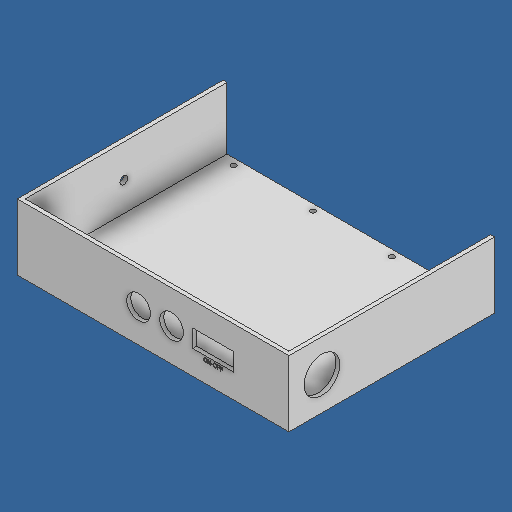
# Autodesk Inventor part: Chasis
Saved by Autodesk Inventor 2025 (Build 290162000, 162)
## iProperties
Created: 2025-09-23
Part Number: Chasis
Material: Genérico
Document SubType Name: Modeling
Designer: HP
Density: 1 g/cm^3
Appearance: Valor por defecto
Author: HP
Autodesk Inventor part; units mm, degrees
ref_plane "YZ Plane" through (0, 0, 0) normal (1, 0, 0) x (0, 1, 0)
ref_plane "XZ Plane" through (0, 0, 0) normal (0, 1, 0) x (-1, 0, 0)
ref_plane "XY Plane" through (0, 0, 0) normal (0, 0, 1) x (1, 0, 0)
sketch "Boceto1" plane through (0, 0, 0) normal (0, 1, 0) x (-1, 0, 0)
  line L0 (-100, 75) -> (100, 75)
  line L1 (100, 75) -> (100, -75)
  line L2 (100, -75) -> (-100, -75)
  line L3 (-100, -75) -> (-100, 75)
  line L4 (-100, 75) -> (100, -75) construction
  line L5 (100, 75) -> (-100, -75) construction
  point P0 (0, 0)
  dimension "d0" = 200
  dimension "d1" = 150
  constraints: 12 end point, 2 midpoint, 2 parallel, 1 horizontal, 1 perpendicular
  measures "d0" distance of L1.end L2.end
  measures "d1" distance of L0.end L1.end
extrude "Extrusión1" add sketch "Boceto1" along normal blind 3
sketch "Boceto2" plane through (0, 0, 0) normal (0, 1, 0) x (-1, 0, 0)
  line L0 (-100, -75) -> (100, -75) projected
  line L1 (100, -75) -> (100, 75) projected
  line L2 (100, 75) -> (-100, 75) projected
  line L3 (-100, 75) -> (-100, -75) projected
  line L4 (103, 78) -> (103, -78)
  line L5 (103, -78) -> (-103, -78)
  line L6 (-103, -78) -> (-103, 78)
  line L7 (-103, 78) -> (103, 78)
  point P0 (0, 0)
  dimension "d4" = 3
  constraints: 8 end point, 3 other
  measures "d4" distance between parallel lines of L1 L4
extrude "Extrusión2" add sketch "Boceto2" along normal blind 50
sketch "Boceto3" plane through (-103, 0, -78) normal (-1, 0, 0) x (0, 0, 1)
  line L0 (78, 0) -> (78, 50) construction
  line L1 (3, 50) -> (153, 50) construction
  line L2 (156, 0) -> (156, 50) construction
  line L3 (156, 25) -> (0.5528, 25) construction
  circle A0 centre (78.2764, 25) radius 3
  line L4 (0, 0) -> (156, 0) projected
  line L5 (156, 0) -> (156, 50) projected
  line L6 (0, 50) -> (156, 50) projected
  line L7 (0, 0) -> (0, 50) projected
  line L8 (0, 0) -> (156, 0) projected
  dimension "d7" = 6
  dimension "d11" = 25
  constraints: 4 end point, 3 midpoint, 1 centre point, 1 horizontal
  measures "d7" diameter of A0
  measures "d11" distance between parallel lines of L4 L3
extrude "Extrusión3" cut sketch "Boceto3" against normal blind 3 contours A0
sketch "Boceto4" plane through (-103, 0, 78) normal (0, 0, 1) x (1, 0, 0)
  line L0 (0, 0) -> (206, 0) projected
  line L1 (0, 25) -> (206, 25)
  circle A0 centre (92, 25) radius 9
  circle A1 centre (117, 25) radius 9
  line L2 (133, 18.25) -> (164, 18.25)
  line L3 (164, 18.25) -> (164, 31.75)
  line L4 (164, 31.75) -> (133, 31.75)
  line L5 (133, 31.75) -> (133, 18.25)
  line L6 (133, 18.25) -> (164, 31.75) construction
  line L7 (164, 18.25) -> (133, 31.75) construction
  line L8 (206, 0) -> (206, 50) projected
  line L9 (141.1134, 17.0625) -> (155.7384, 17.0625) construction
  line L10 (155.7384, 17.0625) -> (155.7384, 13.8861) construction
  line L11 (155.7384, 13.8861) -> (141.1134, 13.8861) construction
  line L12 (141.1134, 13.8861) -> (141.1134, 17.0625) construction
  spline S0 degree 2 poles (143.5785, 16.6501) (143.7514, 16.4475) (143.944, 15.8547) (143.944, 15.4743) knots 0 0 0 1 2 2 2
  spline S1 degree 2 poles (143.944, 15.4743) (143.944, 15.1038) (143.7563, 14.5036) (143.5785, 14.3011) knots 0 0 0 1 2 2 2
  spline S2 degree 2 poles (143.5785, 14.3011) (143.3907, 14.0886) (142.8943, 13.8861) (142.5954, 13.8861) knots 0 0 0 1 2 2 2
  spline S3 degree 2 poles (142.5954, 13.8861) (142.2866, 13.8861) (141.7926, 14.0961) (141.6123, 14.3011) knots 0 0 0 1 2 2 2
  spline S4 degree 2 poles (141.6123, 14.3011) (141.437, 14.5036) (141.2492, 15.0989) (141.2492, 15.4743) knots 0 0 0 1 2 2 2
  spline S5 degree 2 poles (141.2492, 15.4743) (141.2492, 15.8572) (141.4394, 16.4401) (141.6148, 16.6501) knots 0 0 0 1 2 2 2
  spline S6 degree 2 poles (141.6148, 16.6501) (141.7926, 16.8526) (142.2891, 17.0625) (142.5954, 17.0625) knots 0 0 0 1 2 2 2
  spline S7 degree 2 poles (142.5954, 17.0625) (142.9066, 17.0625) (143.4056, 16.8452) (143.5785, 16.6501) knots 0 0 0 1 2 2 2
  spline S8 degree 2 poles (143.5217, 15.4743) (143.5217, 15.7757) (143.3907, 16.2425) (143.2722, 16.3956) knots 0 0 0 1 2 2 2
  spline S9 degree 2 poles (143.2722, 16.3956) (143.1511, 16.5537) (142.8103, 16.7118) (142.5979, 16.7118) knots 0 0 0 1 2 2 2
  spline S10 degree 2 poles (142.5979, 16.7118) (142.378, 16.7118) (142.0471, 16.5587) (141.9211, 16.3956) knots 0 0 0 1 2 2 2
  spline S11 degree 2 poles (141.9211, 16.3956) (141.8, 16.24) (141.6716, 15.7707) (141.6716, 15.4743) knots 0 0 0 1 2 2 2
  spline S12 degree 2 poles (141.6716, 15.4743) (141.6716, 14.8741) (142.1755, 14.2368) (142.5979, 14.2368) knots 0 0 0 1 2 2 2
  spline S13 degree 2 poles (142.5979, 14.2368) (143.0202, 14.2368) (143.5217, 14.8741) (143.5217, 15.4743) knots 0 0 0 1 2 2 2
  line L13 (146.5697, 13.9503) -> (146.1152, 13.9503)
  line L14 (146.1152, 13.9503) -> (144.7665, 16.5784)
  line L15 (144.7665, 16.5784) -> (144.7665, 13.9503)
  line L16 (144.7665, 13.9503) -> (144.3886, 13.9503)
  line L17 (144.3886, 13.9503) -> (144.3886, 16.9983)
  line L18 (144.3886, 16.9983) -> (144.9641, 16.9983)
  line L19 (144.9641, 16.9983) -> (146.1917, 14.5851)
  line L20 (146.1917, 14.5851) -> (146.1917, 16.9983)
  line L21 (146.1917, 16.9983) -> (146.5697, 16.9983)
  line L22 (146.5697, 16.9983) -> (146.5697, 13.9503)
  line L23 (148.2172, 15.0989) -> (147.0637, 15.0989)
  line L24 (147.0637, 15.0989) -> (147.0637, 15.4694)
  line L25 (147.0637, 15.4694) -> (148.2172, 15.4694)
  line L26 (148.2172, 15.4694) -> (148.2172, 15.0989)
  spline S14 degree 2 poles (150.865, 16.6501) (151.0379, 16.4475) (151.2306, 15.8547) (151.2306, 15.4743) knots 0 0 0 1 2 2 2
  spline S15 degree 2 poles (151.2306, 15.4743) (151.2306, 15.1038) (151.0428, 14.5036) (150.865, 14.3011) knots 0 0 0 1 2 2 2
  spline S16 degree 2 poles (150.865, 14.3011) (150.6773, 14.0886) (150.1808, 13.8861) (149.8819, 13.8861) knots 0 0 0 1 2 2 2
  spline S17 degree 2 poles (149.8819, 13.8861) (149.5732, 13.8861) (149.0792, 14.0961) (148.8989, 14.3011) knots 0 0 0 1 2 2 2
  spline S18 degree 2 poles (148.8989, 14.3011) (148.7235, 14.5036) (148.5358, 15.0989) (148.5358, 15.4743) knots 0 0 0 1 2 2 2
  spline S19 degree 2 poles (148.5358, 15.4743) (148.5358, 15.8572) (148.726, 16.4401) (148.9013, 16.6501) knots 0 0 0 1 2 2 2
  spline S20 degree 2 poles (148.9013, 16.6501) (149.0792, 16.8526) (149.5757, 17.0625) (149.8819, 17.0625) knots 0 0 0 1 2 2 2
  spline S21 degree 2 poles (149.8819, 17.0625) (150.1932, 17.0625) (150.6921, 16.8452) (150.865, 16.6501) knots 0 0 0 1 2 2 2
  spline S22 degree 2 poles (150.8082, 15.4743) (150.8082, 15.7757) (150.6773, 16.2425) (150.5587, 16.3956) knots 0 0 0 1 2 2 2
  spline S23 degree 2 poles (150.5587, 16.3956) (150.4377, 16.5537) (150.0968, 16.7118) (149.8844, 16.7118) knots 0 0 0 1 2 2 2
  spline S24 degree 2 poles (149.8844, 16.7118) (149.6646, 16.7118) (149.3336, 16.5587) (149.2076, 16.3956) knots 0 0 0 1 2 2 2
  spline S25 degree 2 poles (149.2076, 16.3956) (149.0866, 16.24) (148.9582, 15.7707) (148.9582, 15.4743) knots 0 0 0 1 2 2 2
  spline S26 degree 2 poles (148.9582, 15.4743) (148.9582, 14.8741) (149.462, 14.2368) (149.8844, 14.2368) knots 0 0 0 1 2 2 2
  spline S27 degree 2 poles (149.8844, 14.2368) (150.3068, 14.2368) (150.8082, 14.8741) (150.8082, 15.4743) knots 0 0 0 1 2 2 2
  line L27 (153.498, 16.6377) -> (152.0803, 16.6377)
  line L28 (152.0803, 16.6377) -> (152.0803, 15.7781)
  line L29 (152.0803, 15.7781) -> (153.4388, 15.7781)
  line L30 (153.4388, 15.7781) -> (153.4388, 15.4175)
  line L31 (153.4388, 15.4175) -> (152.0803, 15.4175)
  line L32 (152.0803, 15.4175) -> (152.0803, 13.9503)
  line L33 (152.0803, 13.9503) -> (151.6752, 13.9503)
  line L34 (151.6752, 13.9503) -> (151.6752, 16.9983)
  line L35 (151.6752, 16.9983) -> (153.498, 16.9983)
  line L36 (153.498, 16.9983) -> (153.498, 16.6377)
  line L37 (155.684, 16.6377) -> (154.2662, 16.6377)
  line L38 (154.2662, 16.6377) -> (154.2662, 15.7781)
  line L39 (154.2662, 15.7781) -> (155.6247, 15.7781)
  line L40 (155.6247, 15.7781) -> (155.6247, 15.4175)
  line L41 (155.6247, 15.4175) -> (154.2662, 15.4175)
  line L42 (154.2662, 15.4175) -> (154.2662, 13.9503)
  line L43 (154.2662, 13.9503) -> (153.8611, 13.9503)
  line L44 (153.8611, 13.9503) -> (153.8611, 16.9983)
  line L45 (153.8611, 16.9983) -> (155.684, 16.9983)
  line L46 (155.684, 16.9983) -> (155.684, 16.6377)
  point P0 (103, 0)
  point P1 (148.5, 25)
  dimension "d0" = 200
  dimension "d1" = 150
  dimension "d10" = 25
  dimension "d12" = 18
  dimension "d13" = 18
  dimension "d14" = 31
  dimension "d15" = 13.5
  dimension "d16" = 42
  dimension "d17" = 25
  dimension "d18" = 16
  constraints: 14 end point, 3 parallel, 3 point on line, 2 centre point, 2 midpoint, 1 horizontal, 1 perpendicular, 2 other
  measures "d10" distance between parallel lines of L0 L1
  measures "d12" diameter of A0
  measures "d13" diameter of A1
  measures "d14" distance of L4.end L3.end
  measures "d15" distance of L3.end L2.end
  measures "d16" distance between parallel lines of L8 L3
  measures "d17" distance of A0.centre A1.centre
  measures "d18" distance from line of A1.centre L5
extrude "Extrusión4" cut sketch "Boceto4" against normal blind 25 contours A0 L1 | L5 L4 L3 L1 | L1 L3 L2 L5 | A1 L1 | L1 A1 | L1 A0
extrude "Extrusión5" cut sketch "Boceto4" against normal blind 2 contours S0 S1 S2 S3 S4 S5 S6 S7 | L13 L14 L15 L16 L17 L18 L19 L20 L21 L22 | L23 L24 L25 L26 | S14 S15 S16 S17 S18 S19 S20 S21 | L27 L28 L29 L30 L31 L32 L33 L34 L35 L36 | L37 L38 L39 L40 L41 L42 L43 L44 L45 L46
sketch "Boceto5" plane through (-100, 3, -75) normal (0, 0, 1) x (1, 0, 0)
  line L0 (200, 0) -> (0, 0) projected
  line L1 (200, 0) -> (200, 47) projected
  line L2 (0, 47) -> (200, 47) projected
  line L3 (0, 0) -> (0, 47) projected
  point P0 (100, -3)
extrude "Extrusión6" cut sketch "Boceto5" against normal blind 3
sketch "Boceto6" plane through (0, 3, 0) normal (0, 1, 0) x (1, 0, 0)
  line L0 (-100, 78) -> (100, 78) projected
  line L1 (-100, 73) -> (100, 73) construction
  circle A0 centre (-90, 73) radius 2
  line L2 (-100, -75) -> (-100, 78) projected
  circle A1 centre (-30, 73) radius 2
  circle A2 centre (30, 73) radius 2
  circle A3 centre (90, 73) radius 2
  point P0 (0, 0)
  dimension "d25" = 5
  dimension "d26" = 4
  dimension "d27" = 10
  dimension "d30" = 60
  constraints: 4 centre point, 2 end point, 1 horizontal, 1 parallel, 1 point on line, 6 other
  measures "d25" distance between parallel lines of L0 L1
  measures "d26" diameter of A0
  measures "d27" distance from line of L2 A0.centre
  measures "d30" distance of A0.centre A1.centre
extrude "Extrusión7" cut sketch "Boceto6" against normal blind 3
sketch "Boceto7" plane through (103, 0, 78) normal (1, 0, 0) x (0, 0, -1)
  line L0 (-0.5059, 25) -> (155.9287, 25) construction
  line L1 (156, 50) -> (3, 50) construction
  line L2 (25, 50) -> (25, 0) construction
  line L3 (0, 0) -> (0, 50) construction
  circle A0 centre (25, 25) radius 13.6
  point P0 (78, 0)
  dimension "d37" = 25
  dimension "d38" = 27.2
  constraints: 4 end point, 1 centre point, 1 horizontal, 1 midpoint, 1 perpendicular, 1 point on line
  measures "d37" distance between parallel lines of L3 L2
  measures "d38" diameter of A0
extrude "Extrusión8" cut sketch "Boceto7" against normal blind 3
equation "\"d19\" = d17"
